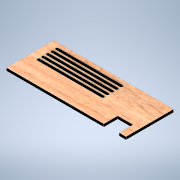
# Autodesk Inventor part: wood_front
Saved by Autodesk Inventor 2021 (Build 250183000, 183)
## iProperties
Created: 2021-08-17
Part Number: wood_front
Material: Generisch
Document SubType Name: Modeling
Designer: Tilman
Density: 1 g/cm^3
Appearance: Eloxiert - Schwarz
Author: Tilman
Autodesk Inventor part; units mm, degrees
ref_plane "YZ Plane" through (0, 0, 0) normal (1, 0, 0) x (0, 1, 0)
ref_plane "XZ Plane" through (0, 0, 0) normal (0, 1, 0) x (-1, 0, 0)
ref_plane "XY Plane" through (0, 0, 0) normal (0, 0, 1) x (1, 0, 0)
sketch "Skizze1" plane through (0, 0, 0) normal (0, 1, 0) x (-1, 0, 0)
  line L0 (0, 0) -> (-129.5, 0)
  line L1 (-129.5, 0) -> (-129.5, -51.5)
  line L2 (-129.5, -51.5) -> (0, -51.5)
  line L3 (0, -51.5) -> (0, 0)
  line L4 (-122, 0) -> (-122, -15)
  line L5 (-122, -15) -> (-105.5, -15)
  line L6 (-105.5, -15) -> (-105.5, 0)
  dimension "d0" = 129.5
  dimension "d1" = 51.5
  dimension "d4" = 16.5
  dimension "d5" = 7.5
  dimension "d6" = 15
  constraints: 14 end point, 3 perpendicular, 2 parallel, 2 point on line, 1 horizontal, 1 vertical
  measures "d0" distance of L0.start L0.end
  measures "d1" distance of L2.end L0.start
  measures "d4" distance of L4.end L5.end
  measures "d5" distance between parallel lines of L1 L4
  measures "d6" distance of L5.end L6.end
extrude "Extrusion1" add sketch "Skizze1" along normal blind 3 contours L3 L2 L1 L0 L4 L5 L6
sketch "Skizze2" plane through (0, 3, 0) normal (0, 1, 0) x (1, 0, 0)
  line L0 (10, 45) -> (79.5, 45) construction
  line L1 (10, 43.5) -> (79.5, 43.5)
  line L2 (79.5, 46.5) -> (10, 46.5)
  arc A0 (10, 46.5) -> (10, 43.5) centre (10, 45) ccw
  arc A1 (79.5, 43.5) -> (79.5, 46.5) centre (79.5, 45) ccw
  line L3 (0, 0) -> (105.5, 0) projected
  line L4 (105.5, 0) -> (105.5, 15) projected
  line L5 (105.5, 15) -> (122, 15) projected
  line L6 (122, 15) -> (122, 0) projected
  line L7 (122, 0) -> (129.5, 0) projected
  line L8 (129.5, 0) -> (129.5, 51.5) projected
  line L9 (129.5, 51.5) -> (0, 51.5) projected
  line L10 (0, 51.5) -> (0, 0) projected
  point P0 (44.75, 45)
  dimension "d7" = 5
  dimension "d8" = 10
  dimension "d9" = 50
  dimension "d10" = 1.5
  constraints: 8 end point, 4 point on circle, 4 tangent, 2 centre point, 1 horizontal, 1 midpoint, 1 parallel
  measures "d7" distance between parallel lines of L9 L2
  measures "d8" distance from line of L10 L0.start
  measures "d9" distance from line of L8 L0.end
  measures "d10" radius of A1
extrude "Extrusion2" cut sketch "Skizze2" against normal through all contours A0 L2 A1 L1
pattern_linear "Rechteckige Anordnung1" count 5 spacing 5 along (0, 0, 1) of "Extrusion2"
